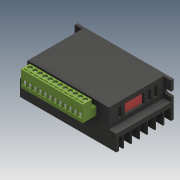
# Autodesk Inventor part: driver WD-2404
Saved by Autodesk Inventor 2017 (Build 210142000, 142)
## iProperties
Created: 2018-07-15
Part Number: driver WD-2404
Material: Aluminum 6061
Document SubType Name: Modeling
Designer: Luiz Gustavo
Density: 2.7 g/cm^3
Appearance: Smooth - Black
Author: Luiz Gustavo
Autodesk Inventor part; units mm, degrees
ref_plane "YZ Plane" through (0, 0, 0) normal (1, 0, 0) x (0, 1, 0)
ref_plane "XZ Plane" through (0, 0, 0) normal (0, 1, 0) x (-1, 0, 0)
ref_plane "XY Plane" through (0, 0, 0) normal (0, 0, 1) x (1, 0, 0)
sketch "Sketch1" plane through (0, 0, 0) normal (0, 0, 1) x (1, 0, 0)
  line L0 (-48, 28.5) -> (48, 28.5)
  line L1 (48, 28.5) -> (48, -28.5)
  line L2 (48, -28.5) -> (-48, -28.5)
  line L3 (-48, -28.5) -> (-48, 28.5)
  line L4 (-48, 28.5) -> (48, -28.5) construction
  line L5 (48, 28.5) -> (-48, -28.5) construction
  point P0 (0, 0)
  dimension "d0" = 96
  dimension "d1" = 57
  constraints: 12 end point, 2 midpoint, 2 parallel, 1 horizontal, 1 perpendicular
  measures "d0" distance of L1.end L2.end
  measures "d1" distance of L0.end L1.end
extrude "Extrusion1" add sketch "Sketch1" along normal blind 35
sketch "Sketch2" plane through (0, 0, 0) normal (0, 0, 1) x (1, 0, 0)
  line L0 (-48, 28.5) -> (48, 28.5) projected
  line L1 (48, 28.5) -> (48, -28.5) projected
  line L2 (48, -28.5) -> (-48, -28.5) projected
  line L3 (-48, -28.5) -> (-48, 28.5) projected
  line L4 (48, -28.5) -> (48, 28.5) projected
  line L5 (-48, 28.5) -> (-48, -28.5) projected
  line L6 (48, 25.8) -> (-48, 25.8)
  line L7 (-48, 25.8) -> (-48, 19)
  line L8 (-48, 19) -> (48, 19)
  line L9 (48, 19) -> (48, 25.8)
  line L10 (48, 17.8) -> (-48, 17.8)
  line L11 (-48, 17.8) -> (-48, 11)
  line L12 (-48, 11) -> (48, 11)
  line L13 (48, 11) -> (48, 17.8)
  line L14 (48, 9.8) -> (-48, 9.8)
  line L15 (-48, 9.8) -> (-48, 3)
  line L16 (-48, 3) -> (48, 3)
  line L17 (48, 3) -> (48, 9.8)
  line L18 (48, 1.8) -> (-48, 1.8)
  line L19 (-48, 1.8) -> (-48, -5)
  line L20 (-48, -5) -> (48, -5)
  line L21 (48, -5) -> (48, 1.8)
  line L22 (48, -6.2) -> (-48, -6.2)
  line L23 (-48, -6.2) -> (-48, -13)
  line L24 (-48, -13) -> (48, -13)
  line L25 (48, -13) -> (48, -6.2)
  line L26 (48, -14.2) -> (-48, -14.2)
  line L27 (-48, -14.2) -> (-48, -21)
  line L28 (-48, -21) -> (48, -21)
  line L29 (48, -21) -> (48, -14.2)
  line L30 (48, -22.2) -> (-48, -22.2)
  line L31 (-48, -22.2) -> (-48, -29)
  line L32 (-48, -29) -> (48, -29)
  line L33 (48, -29) -> (48, -22.2)
  line L34 (48, -25.8) -> (-48, -25.8)
  point P0 (0, 0)
  dimension "d4" = 6.8
  dimension "d5" = 2.7
  dimension "d8" = 8
  dimension "d13" = 2.7
  constraints: 58 end point, 4 point on line, 2 parallel, 2 perpendicular, 1 horizontal, 1 vertical, 48 other
  measures "d4" distance between parallel lines of L8 L6
  measures "d5" distance between parallel lines of L6 L0
  measures "d8" distance of L6.start L10.start
  measures "d13" distance between parallel lines of L2 L34
extrude "Extrusion2" cut sketch "Sketch2" along normal blind 11.6 contours L6 L1 L8 L3 | L10 L1 L12 L3 | L14 L1 L16 L3 | L18 L1 L20 L3 | L22 L1 L24 L3 | L26 L1 L28 L3 | L30 L1 L34 L3
sketch "Sketch3" plane through (0, 0, 35) normal (0, 0, 1) x (1, 0, 0)
  line L0 (48, 28.5) -> (-48, 28.5) projected
  line L1 (-48, 28.5) -> (-48, -28.5) construction
  line L2 (-48, -28.5) -> (48, -28.5) construction
  line L3 (48, -28.5) -> (48, 28.5) construction
  line L4 (-48, -28.5) -> (48, -28.5) projected
  line L5 (-40.5, -28.5) -> (40.5, -28.5)
  line L6 (40.5, -28.5) -> (40.5, 25.8)
  line L7 (40.5, 25.8) -> (-40.5, 25.8)
  line L8 (-40.5, 25.8) -> (-40.5, -28.5)
  line L9 (48, 28.5) -> (-48, 28.5) construction
  line L10 (0, 28.5) -> (0, -28.5) construction
  line L11 (48, 25.8) -> (-48, 25.8) construction
  line L12 (48, 25.8) -> (-48, 25.8) projected
  line L13 (-48, 25.8) -> (-40.5, 25.8)
  line L14 (40.5, 25.8) -> (48, 25.8)
  line L15 (-48, 25.8) -> (-48, -28.5)
  line L16 (48, -28.5) -> (48, 28.5) projected
  line L17 (48, 25.8) -> (48, -28.5)
  line L18 (48, -28.5) -> (40.5, -28.5)
  line L19 (-48, -28.5) -> (-40.5, -28.5)
  point P0 (0, 0)
  dimension "d16" = 81
  constraints: 22 end point, 5 collinear, 2 midpoint, 2 parallel, 2 perpendicular, 1 horizontal, 1 point on line, 1 vertical, 1 other
  measures "d16" distance between parallel lines of L6 L8
extrude "Extrusion3" cut sketch "Sketch3" against normal blind 19 contours L15 L12 L8 L4 | L6 L12 L16 L4
sketch "Sketch4" plane through (-48, 28.5, 0) normal (0, 1, 0) x (1, 0, 0)
  line L0 (0, 0) -> (96, 0) projected
  line L1 (0, 0) -> (0, -35) projected
  line L2 (96, -35) -> (0, -35) projected
  line L3 (96, 0) -> (96, -35) projected
  line L4 (96, -35) -> (96, -16) construction
  line L5 (0, -16) -> (0, -35) construction
  line L6 (96, -23) -> (0, -23) construction
  arc A0 (91, -25.25) -> (91, -20.75) centre (91, -23) ccw construction
  line L7 (91, -25.25) -> (96, -25.25)
  line L8 (91, -20.75) -> (96, -20.75)
  line L9 (96, -25.25) -> (96, -20.75)
  arc A1 (88.75, -23) -> (91, -25.25) centre (91, -23) ccw
  arc A2 (91, -20.75) -> (88.75, -23) centre (91, -23) ccw
  line L10 (48, 0) -> (48, -35) construction
  arc A3 (5, -20.75) -> (5, -25.25) centre (5, -23) ccw construction
  line L11 (5, -25.25) -> (0, -25.25)
  line L12 (5, -20.75) -> (0, -20.75)
  line L13 (0, -25.25) -> (0, -20.75)
  arc A4 (5, -25.25) -> (7.25, -23) centre (5, -23) ccw
  arc A5 (7.25, -23) -> (5, -20.75) centre (5, -23) ccw
  dimension "d21" = 12
  dimension "d22" = 4.5
  dimension "d23" = 5
  constraints: 16 end point, 12 point on circle, 6 centre point, 6 point on line, 6 symmetric about line, 4 tangent, 3 horizontal, 1 midpoint, 1 vertical, 3 other
  measures "d21" distance between parallel lines of L6 L2
  measures "d22" diameter of A0
  measures "d23" distance of L7.start L7.end
extrude "Extrusion4" cut sketch "Sketch4" against normal through all contours L12 A5 A4 L11 L1 | L3 L7 A1 A2 L8
sketch "Sketch5" plane through (-48, -28.5, 0) normal (0, -1, 0) x (1, 0, 0)
  line L0 (14.5, 30) -> (76, 30)
  line L1 (76, 30) -> (76, 22)
  line L2 (76, 22) -> (14.5, 22)
  line L3 (14.5, 22) -> (14.5, 30)
  line L4 (7.5, 35) -> (7.5, 16) projected
  line L5 (7.5, 35) -> (88.5, 35) projected
  point P0 (48, 0)
  dimension "d26" = 61.5
  dimension "d27" = 8
  dimension "d28" = 7
  dimension "d29" = 5
  constraints: 8 end point, 2 parallel, 1 horizontal, 1 perpendicular
  measures "d26" distance of L1.end L2.end
  measures "d27" distance of L0.end L1.end
  measures "d28" distance between parallel lines of L4 L3
  measures "d29" distance between parallel lines of L0 L5
extrude "Extrusion5" add sketch "Sketch5" along normal blind 13.6
sketch "Sketch6" plane through (-33.5, -28.5, 30) normal (0, 0, 1) x (1, 0, 0)
  line L0 (0, 0) -> (61.5, 0) projected
  line L1 (0, 0) -> (0, -13.6) projected
  line L2 (61.5, -13.6) -> (0, -13.6) projected
  line L3 (61.5, 0) -> (61.5, -13.6) projected
  line L4 (61.5, -13.6) -> (0, -13.6)
  line L5 (0, -13.6) -> (0, -4.6)
  line L6 (0, -4.6) -> (61.5, -4.6)
  line L7 (61.5, -4.6) -> (61.5, -13.6)
  line L8 (0, 0) -> (0, -13.6) projected
  point P0 (33.5, 28.5)
  dimension "d32" = 9
  constraints: 8 end point, 2 parallel, 1 horizontal, 1 perpendicular, 1 point on line
  measures "d32" distance between parallel lines of L6 L4
extrude "Extrusion6" add sketch "Sketch6" along normal blind 8 contours L6 L3 L2 L1
sketch "Sketch7" plane through (-33.5, -28.5, 38) normal (0, 0, 1) x (1, 0, 0)
  line L0 (0, -4.6) -> (0, -13.6) projected
  line L1 (0, -13.6) -> (61.5, -13.6) projected
  line L2 (61.5, -13.6) -> (61.5, -4.6) projected
  line L3 (61.5, -4.6) -> (0, -4.6) projected
  circle A0 centre (58.25, -7.6) radius 2
  line L4 (60.25, -11.2) -> (56.25, -11.2)
  line L5 (56.25, -11.2) -> (56.25, -12.4)
  line L6 (56.25, -12.4) -> (60.25, -12.4)
  line L7 (60.25, -12.4) -> (60.25, -11.2)
  line L8 (60.25, -11.2) -> (60.25, -7.6) construction
  line L9 (56.25, -11.2) -> (56.25, -7.6) construction
  circle A1 centre (53.25, -7.6) radius 2
  line L10 (55.25, -11.2) -> (51.25, -11.2)
  line L11 (55.25, -12.4) -> (55.25, -11.2)
  line L12 (51.25, -12.4) -> (55.25, -12.4)
  line L13 (51.25, -11.2) -> (51.25, -12.4)
  circle A2 centre (48.25, -7.6) radius 2
  line L14 (50.25, -11.2) -> (46.25, -11.2)
  line L15 (50.25, -12.4) -> (50.25, -11.2)
  line L16 (46.25, -12.4) -> (50.25, -12.4)
  line L17 (46.25, -11.2) -> (46.25, -12.4)
  circle A3 centre (43.25, -7.6) radius 2
  line L18 (45.25, -11.2) -> (41.25, -11.2)
  line L19 (45.25, -12.4) -> (45.25, -11.2)
  line L20 (41.25, -12.4) -> (45.25, -12.4)
  line L21 (41.25, -11.2) -> (41.25, -12.4)
  circle A4 centre (38.25, -7.6) radius 2
  line L22 (40.25, -11.2) -> (36.25, -11.2)
  line L23 (40.25, -12.4) -> (40.25, -11.2)
  line L24 (36.25, -12.4) -> (40.25, -12.4)
  line L25 (36.25, -11.2) -> (36.25, -12.4)
  circle A5 centre (33.25, -7.6) radius 2
  line L26 (35.25, -11.2) -> (31.25, -11.2)
  line L27 (35.25, -12.4) -> (35.25, -11.2)
  line L28 (31.25, -12.4) -> (35.25, -12.4)
  line L29 (31.25, -11.2) -> (31.25, -12.4)
  circle A6 centre (28.25, -7.6) radius 2
  line L30 (30.25, -11.2) -> (26.25, -11.2)
  line L31 (30.25, -12.4) -> (30.25, -11.2)
  line L32 (26.25, -12.4) -> (30.25, -12.4)
  line L33 (26.25, -11.2) -> (26.25, -12.4)
  circle A7 centre (23.25, -7.6) radius 2
  line L34 (25.25, -11.2) -> (21.25, -11.2)
  line L35 (25.25, -12.4) -> (25.25, -11.2)
  line L36 (21.25, -12.4) -> (25.25, -12.4)
  line L37 (21.25, -11.2) -> (21.25, -12.4)
  circle A8 centre (18.25, -7.6) radius 2
  line L38 (20.25, -11.2) -> (16.25, -11.2)
  line L39 (20.25, -12.4) -> (20.25, -11.2)
  line L40 (16.25, -12.4) -> (20.25, -12.4)
  line L41 (16.25, -11.2) -> (16.25, -12.4)
  circle A9 centre (13.25, -7.6) radius 2
  line L42 (15.25, -11.2) -> (11.25, -11.2)
  line L43 (15.25, -12.4) -> (15.25, -11.2)
  line L44 (11.25, -12.4) -> (15.25, -12.4)
  line L45 (11.25, -11.2) -> (11.25, -12.4)
  circle A10 centre (8.25, -7.6) radius 2
  line L46 (10.25, -11.2) -> (6.25, -11.2)
  line L47 (10.25, -12.4) -> (10.25, -11.2)
  line L48 (6.25, -12.4) -> (10.25, -12.4)
  line L49 (6.25, -11.2) -> (6.25, -12.4)
  circle A11 centre (3.25, -7.6) radius 2
  line L50 (5.25, -11.2) -> (1.25, -11.2)
  line L51 (5.25, -12.4) -> (5.25, -11.2)
  line L52 (1.25, -12.4) -> (5.25, -12.4)
  line L53 (1.25, -11.2) -> (1.25, -12.4)
  point P0 (33.5, 28.5)
  point P1 (55.25, -7.6)
  point P2 (51.25, -7.6)
  point P3 (50.25, -7.6)
  point P4 (46.25, -7.6)
  point P5 (45.25, -7.6)
  point P6 (41.25, -7.6)
  point P7 (40.25, -7.6)
  point P8 (36.25, -7.6)
  point P9 (35.25, -7.6)
  point P10 (31.25, -7.6)
  point P11 (30.25, -7.6)
  point P12 (26.25, -7.6)
  point P13 (25.25, -7.6)
  point P14 (21.25, -7.6)
  point P15 (20.25, -7.6)
  point P16 (16.25, -7.6)
  point P17 (15.25, -7.6)
  point P18 (11.25, -7.6)
  point P19 (10.25, -7.6)
  point P20 (6.25, -7.6)
  point P21 (5.25, -7.6)
  point P22 (1.25, -7.6)
  dimension "d35" = 4
  dimension "d36" = 1.2
  dimension "d37" = 1.2
  dimension "d38" = 3
  dimension "d39" = 3.25
  dimension "d42" = 5
  dimension "d47" = 3.25
  constraints: 100 end point, 24 point on circle, 12 centre point, 2 horizontal, 2 parallel, 2 tangent, 2 vertical, 1 perpendicular, 132 other
  measures "d35" diameter of A0
  measures "d36" distance of L6.end L4.start
  measures "d37" distance between parallel lines of L6 L1
  measures "d38" distance from line of L3 A0.centre
  measures "d39" distance from line of L2 A0.centre
  measures "d42" distance of A0.centre A1.centre
  measures "d47" distance from line of L0 A11.centre
extrude "Extrusion7" cut sketch "Sketch7" against normal blind 2 contours A0 | L7 L6 L5 L4 | A1 | L11 L12 L13 L10 | A2 | L15 L16 L17 L14 | A3 | L19 L20 L21 L18 | A4 | L23 L24 L25 L22 | A5 | L27 L28 L29 L26 | A6 | L31 L32 L33 L30 | A7 | L35 L36 L37 L34 | A8 | L39 L40 L41 L38 | A9 | L43 L44 L45 L42 | A10 | L47 L48 L49 L46 | A11 | L51 L52 L53 L50
sketch "Sketch8" plane through (-48, -42.1, 0) normal (0, -1, 0) x (1, 0, 0)
  line L0 (14.5, 22) -> (14.5, 38) projected
  line L1 (14.5, 22) -> (76, 22) projected
  line L2 (76, 22) -> (76, 38) projected
  line L3 (14.5, 38) -> (76, 38) projected
  line L4 (74.75, 30) -> (70.75, 30)
  line L5 (70.75, 30) -> (70.75, 25)
  line L6 (70.75, 25) -> (74.75, 25)
  line L7 (74.75, 25) -> (74.75, 30)
  line L8 (72.75, 30) -> (72.75, 25) construction
  line L9 (69.75, 30) -> (65.75, 30)
  line L10 (69.75, 25) -> (69.75, 30)
  line L11 (65.75, 25) -> (69.75, 25)
  line L12 (65.75, 30) -> (65.75, 25)
  line L13 (64.75, 30) -> (60.75, 30)
  line L14 (64.75, 25) -> (64.75, 30)
  line L15 (60.75, 25) -> (64.75, 25)
  line L16 (60.75, 30) -> (60.75, 25)
  line L17 (59.75, 30) -> (55.75, 30)
  line L18 (59.75, 25) -> (59.75, 30)
  line L19 (55.75, 25) -> (59.75, 25)
  line L20 (55.75, 30) -> (55.75, 25)
  line L21 (54.75, 30) -> (50.75, 30)
  line L22 (54.75, 25) -> (54.75, 30)
  line L23 (50.75, 25) -> (54.75, 25)
  line L24 (50.75, 30) -> (50.75, 25)
  line L25 (49.75, 30) -> (45.75, 30)
  line L26 (49.75, 25) -> (49.75, 30)
  line L27 (45.75, 25) -> (49.75, 25)
  line L28 (45.75, 30) -> (45.75, 25)
  line L29 (44.75, 30) -> (40.75, 30)
  line L30 (44.75, 25) -> (44.75, 30)
  line L31 (40.75, 25) -> (44.75, 25)
  line L32 (40.75, 30) -> (40.75, 25)
  line L33 (39.75, 30) -> (35.75, 30)
  line L34 (39.75, 25) -> (39.75, 30)
  line L35 (35.75, 25) -> (39.75, 25)
  line L36 (35.75, 30) -> (35.75, 25)
  line L37 (34.75, 30) -> (30.75, 30)
  line L38 (34.75, 25) -> (34.75, 30)
  line L39 (30.75, 25) -> (34.75, 25)
  line L40 (30.75, 30) -> (30.75, 25)
  line L41 (29.75, 30) -> (25.75, 30)
  line L42 (29.75, 25) -> (29.75, 30)
  line L43 (25.75, 25) -> (29.75, 25)
  line L44 (25.75, 30) -> (25.75, 25)
  line L45 (24.75, 30) -> (20.75, 30)
  line L46 (24.75, 25) -> (24.75, 30)
  line L47 (20.75, 25) -> (24.75, 25)
  line L48 (20.75, 30) -> (20.75, 25)
  line L49 (19.75, 30) -> (15.75, 30)
  line L50 (19.75, 25) -> (19.75, 30)
  line L51 (15.75, 25) -> (19.75, 25)
  line L52 (15.75, 30) -> (15.75, 25)
  point P0 (48, 0)
  point P1 (67.75, 30)
  point P2 (67.75, 25)
  point P3 (62.75, 30)
  point P4 (62.75, 25)
  point P5 (57.75, 30)
  point P6 (57.75, 25)
  point P7 (52.75, 30)
  point P8 (52.75, 25)
  point P9 (47.75, 30)
  point P10 (47.75, 25)
  point P11 (42.75, 30)
  point P12 (42.75, 25)
  point P13 (37.75, 30)
  point P14 (37.75, 25)
  point P15 (32.75, 30)
  point P16 (32.75, 25)
  point P17 (27.75, 30)
  point P18 (27.75, 25)
  point P19 (22.75, 30)
  point P20 (22.75, 25)
  point P21 (17.75, 30)
  point P22 (17.75, 25)
  dimension "d50" = 4
  dimension "d51" = 5
  dimension "d52" = 3
  dimension "d54" = 3.25
  dimension "d57" = 5
  constraints: 98 end point, 2 horizontal, 2 midpoint, 2 parallel, 1 perpendicular, 110 other
  measures "d50" distance between parallel lines of L5 L7
  measures "d51" distance of L6.end L4.start
  measures "d52" distance between parallel lines of L6 L1
  measures "d54" distance between parallel lines of L2 L8
  measures "d57" distance of L4.start L9.start
extrude "Extrusion8" cut sketch "Sketch8" against normal blind 2 contours L7 L6 L5 L4 | L10 L11 L12 L9 | L14 L15 L16 L13 | L18 L19 L20 L17 | L22 L23 L24 L21 | L26 L27 L28 L25 | L30 L31 L32 L29 | L34 L35 L36 L33 | L38 L39 L40 L37 | L42 L43 L44 L41 | L46 L47 L48 L45 | L50 L51 L52 L49
sketch "Sketch9" plane through (-40.5, -28.5, 35) normal (-1, 0, 0) x (0, 0, 1)
  line L0 (0, 54.3) -> (0, 0) projected
  line L1 (0, 54.3) -> (-19, 54.3) projected
  line L2 (-19, 54.3) -> (-19, 0) projected
  line L3 (0, 0) -> (-19, 0) projected
  line L4 (-4.5, 47.3) -> (-14.5, 47.3)
  line L5 (-14.5, 47.3) -> (-14.5, 44.3)
  line L6 (-14.5, 44.3) -> (-4.5, 44.3)
  line L7 (-4.5, 44.3) -> (-4.5, 47.3)
  line L8 (0, 0) -> (-19, 0) projected
  line L9 (-9.5, 0) -> (-9.5, 54.3) construction
  line L10 (-4.5, 40.8) -> (-14.5, 40.8)
  line L11 (-14.5, 40.8) -> (-14.5, 37.8)
  line L12 (-14.5, 37.8) -> (-4.5, 37.8)
  line L13 (-4.5, 37.8) -> (-4.5, 40.8)
  line L14 (-4.5, 34.3) -> (-14.5, 34.3)
  line L15 (-14.5, 34.3) -> (-14.5, 31.3)
  line L16 (-14.5, 31.3) -> (-4.5, 31.3)
  line L17 (-4.5, 31.3) -> (-4.5, 34.3)
  line L18 (-4.5, 27.8) -> (-14.5, 27.8)
  line L19 (-14.5, 27.8) -> (-14.5, 24.8)
  line L20 (-14.5, 24.8) -> (-4.5, 24.8)
  line L21 (-4.5, 24.8) -> (-4.5, 27.8)
  line L22 (-4.5, 21.3) -> (-14.5, 21.3)
  line L23 (-14.5, 21.3) -> (-14.5, 18.3)
  line L24 (-14.5, 18.3) -> (-4.5, 18.3)
  line L25 (-4.5, 18.3) -> (-4.5, 21.3)
  line L26 (-4.5, 14.8) -> (-14.5, 14.8)
  line L27 (-14.5, 14.8) -> (-14.5, 11.8)
  line L28 (-14.5, 11.8) -> (-4.5, 11.8)
  line L29 (-4.5, 11.8) -> (-4.5, 14.8)
  line L30 (-4.5, 8.3) -> (-14.5, 8.3)
  line L31 (-14.5, 8.3) -> (-14.5, 5.3)
  line L32 (-14.5, 5.3) -> (-4.5, 5.3)
  line L33 (-4.5, 5.3) -> (-4.5, 8.3)
  point P0 (-35, 28.5)
  dimension "d64" = 10
  dimension "d65" = 3
  dimension "d66" = 7
  dimension "d69" = 6.5
  constraints: 58 end point, 2 midpoint, 2 parallel, 2 vertical, 1 horizontal, 1 perpendicular, 49 other
  measures "d64" distance of L6.end L5.end
  measures "d65" distance of L5.end L4.end
  measures "d66" distance between parallel lines of L1 L4
  measures "d69" distance of L4.start L10.start
extrude "Extrusion9" cut sketch "Sketch9" against normal blind 2 contours L7 L6 L5 L4 | L13 L12 L11 L10 | L17 L16 L15 L14 | L21 L20 L19 L18 | L25 L24 L23 L22 | L29 L28 L27 L26 | L33 L32 L31 L30
sketch "Sketch10" plane through (40.5, -28.5, 35) normal (1, 0, 0) x (0, 0, -1)
  line L0 (0, 0) -> (0, 54.3) projected
  line L1 (19, 0) -> (0, 0) projected
  line L2 (19, 0) -> (19, 54.3) projected
  line L3 (0, 54.3) -> (19, 54.3) projected
  line L4 (4.5, 16) -> (14.5, 16)
  line L5 (14.5, 16) -> (14.5, 35)
  line L6 (14.5, 35) -> (4.5, 35)
  line L7 (4.5, 35) -> (4.5, 16)
  line L8 (0, 0) -> (19, 0) construction
  line L9 (9.5, 0) -> (9.5, 54.3) construction
  line L10 (4.5, 9.5) -> (14.5, 9.5)
  line L11 (14.5, 9.5) -> (14.5, 12.5)
  line L12 (14.5, 12.5) -> (4.5, 12.5)
  line L13 (4.5, 12.5) -> (4.5, 9.5)
  line L14 (4.5, 38.5) -> (14.5, 38.5)
  line L15 (14.5, 38.5) -> (14.5, 41.5)
  line L16 (14.5, 41.5) -> (4.5, 41.5)
  line L17 (4.5, 41.5) -> (4.5, 38.5)
  line L18 (4.5, 45) -> (14.5, 45)
  line L19 (14.5, 45) -> (14.5, 48)
  line L20 (14.5, 48) -> (4.5, 48)
  line L21 (4.5, 48) -> (4.5, 45)
  point P0 (35, 28.5)
  dimension "d76" = 10
  dimension "d77" = 19
  dimension "d78" = 16
  dimension "d79" = 10
  dimension "d80" = 3
  dimension "d81" = 6.5
  dimension "d82" = 6.5
  dimension "d83" = 6.5
  constraints: 34 end point, 8 parallel, 4 equal length, 4 horizontal, 4 perpendicular, 2 midpoint, 4 other
  measures "d76" distance between parallel lines of L5 L7
  measures "d77" distance between parallel lines of L4 L6
  measures "d78" distance between parallel lines of L1 L4
  measures "d79" distance between parallel lines of L11 L13
  measures "d80" distance of L12.end L10.start
  measures "d81" distance between parallel lines of L10 L4
  measures "d82" distance between parallel lines of L16 L20
  measures "d83" distance between parallel lines of L6 L16
extrude "Extrusion10" cut sketch "Sketch10" against normal blind 2 contours L7 L6 L5 L4 | L13 L12 L11 L10 | L17 L16 L15 L14 | L21 L20 L19 L18
equation "\"d13\" = d5"
equation "\"d37\" = d36"
equation "\"d82\" = d81"
equation "\"d83\" = d82"
body "Solid1"
